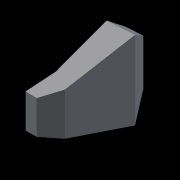
# Autodesk Inventor part: DistalPhalangeIndexMiddle
Saved by Autodesk Inventor 2015 (Build 190159000, 159)
## iProperties
Created: 2014-10-29
Part Number: DistalPhalangeIndexMiddle
Material: Generic
Document SubType Name: Modeling
Designer: Val
Density: 1 g/cm^3
Appearance: Default
Mass: 0.708733 g
Surface Area: 5.61371 cm^2
Volume: 0.708733 cm^3
RuleStatus: InUse
BeforeDocSave0: UpdateBoundingBox
CX: 5.00 mm
CY: 18.00 mm
CZ: 14.00 mm
Author: Val
Autodesk Inventor part; units mm, degrees
ref_plane "YZ Plane" through (0, 0, 0) normal (1, 0, 0) x (0, 1, 0)
ref_plane "XZ Plane" through (0, 0, 0) normal (0, 1, 0) x (-1, 0, 0)
ref_plane "XY Plane" through (0, 0, 0) normal (0, 0, 1) x (1, 0, 0)
sketch "Base" plane through (0, 0, 0) normal (0, 0, 1) x (1, 0, 0)
  line L0 (0, 0) -> (0, -18) construction
  line L1 (0, -18) -> (2, -18)
  line L2 (2, -18) -> (4, -14.9841)
  line L3 (5, -3.4641) -> (3, 0)
  line L4 (3, 0) -> (0, 0)
  line L5 (4, -14.9841) -> (5, -3.4641)
  line L6 (0, -18) -> (0.8747, -13.5)
  line L7 (0.8747, -13.5) -> (0, 0)
  dimension "d0" = 18
  dimension "d1" = 3
  dimension "d2" = 2
  dimension "d3" = 5
  dimension "d8" = 4
  dimension "d12" = 120
  dimension "d14" = 11.52
  dimension "d23" = 13.5
  dimension "d24" = 79
  constraints: 16 end point, 1 parallel, 1 perpendicular, 1 vertical
  measures "d0" distance of L0.start L0.end
  measures "d1" distance of L3.end L0.start
  measures "d2" distance of L0.end L1.end
  measures "d3" distance from line of L3.start L0
  measures "d8" distance from line of L2.end L0
  measures "d12" angle of L3 L4
  measures "d14" vertical distance of L2.end L3.start
  measures "d23" vertical distance of L6.end L0.start
  measures "d24" angle of L6 L1
extrude "BaseFeature" add sketch "Base" along normal blind 14
sketch "TopProfile" plane through (0.8747, -13.5, 0) normal (-0.9979, -0.0647, 0) x (0, 0, 1)
  line L0 (0, 9.7482) -> (14, 9.7482) projected
  line L1 (3, 13.5283) -> (11, 13.5283)
  line L2 (11, 13.5283) -> (14, 9.7482)
  line L3 (14, 9.7482) -> (10, -4.5633)
  line L4 (10, -4.5633) -> (4, -4.5633)
  line L5 (4, -4.5633) -> (0, 9.7482)
  line L6 (0, 9.7482) -> (3, 13.5283)
  line L7 (0, 13.5283) -> (14, 13.5283) projected
  line L8 (0, -4.5633) -> (14, -4.5633) projected
  point P0 (7, 13.5283)
  point P1 (7, -4.5633)
  dimension "d27" = 8
  dimension "d28" = 6
  constraints: 12 end point, 4 midpoint, 2 collinear, 1 horizontal, 1 parallel
  measures "d27" distance of L1.end L1.start
  measures "d28" distance of L3.end L4.end
extrude "TopProfileFeature" cut sketch "TopProfile" along normal through all both and the other way through all keep common part
equation "\"d14\" = 0.64 * d0"
equation "\"d23\" = 0.75 * d0"
